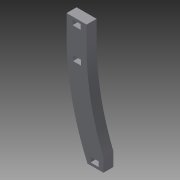
# Autodesk Inventor part: HopperFrontSupport_v2
Saved by Autodesk Inventor 2013 (Build 170138000, 138)
## iProperties
Created: 2013-01-16
Part Number: HopperFrontSupport_v2
Material: Generic
Document SubType Name: Modeling
Designer: twsass
Density: 1 g/cm^3
Mass: 47.1863 g
Surface Area: 132.222 cm^2
Volume: 47.1863 cm^3
Author: twsass
Autodesk Inventor part; units mm, degrees
ref_plane "YZ Plane" through (0, 0, 0) normal (1, 0, 0) x (0, 1, 0)
ref_plane "XZ Plane" through (0, 0, 0) normal (0, 1, 0) x (-1, 0, 0)
ref_plane "XY Plane" through (0, 0, 0) normal (0, 0, 1) x (1, 0, 0)
sketch "Sketch1" plane through (0, 0, 0) normal (0, 0, 1) x (1, 0, 0)
  circle A0 centre (0, 0) radius 292.1
  line L0 (-292.1, 0) -> (-266.7, 0)
  line L1 (-292.1, 0) -> (-317.5, 0)
  circle A1 centre (0, 0) radius 317.5
  line L2 (-317.5, 0) -> (-317.5, -127)
  line L3 (-317.5, -127) -> (-263.0464, -127)
  circle A2 centre (0, 0) radius 317.5
  dimension "d0" = 584.2
  dimension "d1" = 25.4
  dimension "d2" = 25.4
  dimension "d3" = 127
  constraints: 8 end point, 3 coincident, 2 centre point, 2 perpendicular, 2 point on circle, 1 collinear, 1 horizontal, 1 horizontal alignment, 1 vertical, 2 other
  measures "d0" diameter of A0
  measures "d1" distance of L0.start L0.end
  measures "d2" distance of L0.start L1.end
  measures "d3" distance of L1.end L2.end
extrude "Extrusion1" add sketch "Sketch1" along normal blind 12.7 contours A0 L3 A1 L1 | A1 L3 L2 picked at (-275.2864, -120.3141)
sketch "Sketch2" plane through (0, 0, 12.7) normal (0, 0, 1) x (1, 0, 0)
  line L0 (-317.5, 0) -> (-317.5, -127) projected
  line L1 (-317.5, -127) -> (-263.0464, -127) projected
  arc A0 (-292.1, 0) -> (-263.0464, -127) centre (0, 0) ccw projected
  circle A1 centre (0, 0) radius 292.1
  circle A2 centre (0, 0) radius 317.5
  line L2 (-317.5, 0) -> (-317.5, -127)
  line L3 (-317.5, -127) -> (-290.9936, -127)
  constraints: 4 end point, 2 centre point, 2 coincident, 2 point on circle, 1 collinear, 1 concentric, 1 point on line, 1 tangent
extrude "Extrusion2" cut sketch "Sketch2" against normal blind 25.4 contours A2 L1 L0
sketch "Sketch3" plane through (0, 0, 12.7) normal (0, 0, 1) x (1, 0, 0)
  arc A0 (-317.5, 0) -> (-290.9936, -127) centre (0, 0) ccw projected
  line L0 (-290.9936, -127) -> (-316.1859, -127)
  line L1 (-295.9122, -115.0749) -> (-295.9122, -127)
  line L2 (-281.9422, -117.475) -> (-276.8622, -117.475)
  line L3 (-276.8622, -117.475) -> (-276.8622, -123.825)
  line L4 (-276.8622, -123.825) -> (-287.0222, -123.825)
  line L5 (-287.0222, -123.825) -> (-287.0222, -117.475)
  line L6 (-287.0222, -117.475) -> (-281.9422, -117.475)
  line L7 (-290.9936, -127) -> (-263.0464, -127) projected
  dimension "d16" = 5.08
  dimension "d17" = 6.35
  dimension "d18" = 10.16
  dimension "d20" = 4.9186
  dimension "d33" = 13.97
  dimension "d34" = 9.525
  dimension "d35" = 8.89
  constraints: 14 end point, 2 perpendicular, 1 collinear, 1 parallel, 1 point on circle, 1 point on line
  measures "d16" distance of L2.start L2.end
  measures "d17" distance of L2.end L3.end
  measures "d18" distance of L3.end L4.end
  measures "d20" distance from line of L0.start L1
  measures "d33" distance from line of L1 L2.start
  measures "d34" distance between parallel lines of L7 L6
  measures "d35" distance between parallel lines of L1 L5
extrude "Extrusion3" cut sketch "Sketch3" against normal blind 25.4
sketch "Sketch4" plane through (0, 0, 12.7) normal (0, 0, 1) x (1, 0, 0)
  arc A0 (-317.5, 0) -> (-290.9936, -127) centre (0, 0) ccw projected
  arc A1 (-292.1, 0) -> (-263.0464, -127) centre (0, 0) ccw projected
  line L0 (-292.1, 0) -> (-317.5, 0) projected
  line L1 (-317.5, 0) -> (-317.5, 25.4)
  line L2 (-317.5, 25.4) -> (-292.1, 25.4)
  line L3 (-292.1, 25.4) -> (-292.1, 0)
  line L4 (-317.5, 0) -> (-292.1, 0)
  dimension "d24" = 25.4
  constraints: 8 end point, 3 perpendicular, 2 tangent, 1 parallel
  measures "d24" distance of L0.end L1.end
extrude "Extrusion4" add sketch "Sketch4" against normal blind 12.7
sketch "Sketch5" plane through (0, 0, 12.7) normal (0, 0, 1) x (1, 0, 0)
  line L0 (-292.1, 0) -> (-292.1, 25.4) projected
  line L1 (-292.1, 25.4) -> (-317.5, 25.4) projected
  line L2 (-317.5, 25.4) -> (-317.5, 0) projected
  line L3 (-304.8, 25.4) -> (-304.8, 22.225)
  line L4 (-304.8, 22.225) -> (-299.72, 22.225)
  line L5 (-299.72, 22.225) -> (-299.72, 15.875)
  line L6 (-299.72, 15.875) -> (-309.88, 15.875)
  line L7 (-309.88, 15.875) -> (-309.88, 22.225)
  line L8 (-309.88, 22.225) -> (-304.8, 22.225)
  dimension "d27" = 3.175
  dimension "d28" = 5.08
  dimension "d29" = 6.35
  dimension "d30" = 10.16
  constraints: 12 end point, 3 parallel, 3 perpendicular, 1 midpoint
  measures "d27" distance of L3.start L3.end
  measures "d28" distance of L3.end L4.end
  measures "d29" distance of L4.end L5.end
  measures "d30" distance of L5.end L6.end
extrude "Extrusion5" cut sketch "Sketch5" against normal blind 254
sketch "Sketch6" plane through (0, 0, 12.7) normal (0, 0, 1) x (1, 0, 0)
  line L0 (-290.9936, -127) -> (-263.0464, -127) projected
  arc A0 (-292.1, 0) -> (-263.0464, -127) centre (0, 0) ccw projected
  line L1 (-290.9936, -127) -> (-270.6736, -127)
  line L2 (-270.6736, -127) -> (-270.6736, -109.81)
  line L3 (-270.6736, -109.81) -> (-256.8603, -109.81)
  line L4 (-256.8603, -109.81) -> (-256.8603, -127)
  line L5 (-256.8603, -127) -> (-270.6736, -127)
  dimension "d36" = 20.32
  dimension "d37" = 13.8133
  constraints: 10 end point, 3 perpendicular, 1 parallel, 1 point on circle, 1 point on line
  measures "d36" distance of L0.start L1.end
  measures "d37" distance between parallel lines of L2 L4
extrude "Extrusion6" cut sketch "Sketch6" against normal blind 254 contours L2 A0 L0
sketch "Sketch7" plane through (0, 0, 12.7) normal (0, 0, 1) x (1, 0, 0)
  arc A0 (-317.5, 0) -> (-290.9936, -127) centre (0, 0) ccw projected
  line L0 (-276.8622, -117.475) -> (-276.8622, -123.825) projected
  line L1 (-317.5, 0) -> (-317.5, -127) construction
  line L2 (-317.5, -63.5) -> (-317.5, -50.8) construction
  line L3 (-317.5, -50.8) -> (-317.5, -38.1) construction
  line L4 (-317.5, -38.1) -> (-317.5, -25.4) construction
  line L5 (-317.5, -25.4) -> (-317.5, -12.7) construction
  line L6 (-317.5, 23.7649) -> (-317.5, -16.9672) construction
  line L7 (-317.5, -16.9672) -> (-180.5967, -16.9672) construction
  line L8 (-317.5, -16.9672) -> (-309.2958, -16.9672) construction
  line L9 (-309.2958, -16.9672) -> (-309.2958, -23.3172)
  line L10 (-309.2958, -23.3172) -> (-299.1358, -23.3172)
  line L11 (-299.1358, -23.3172) -> (-299.1358, -16.9672)
  line L12 (-309.2958, -16.9672) -> (-299.1358, -16.9672)
  point P0 (-317.5, 25.4)
  dimension "d59" = 8.2042
  dimension "d60" = 6.35
  dimension "d61" = 10.16
  dimension "d65" = 42.3672
  constraints: 24 end point, 7 point on line, 3 perpendicular, 2 parallel, 1 collinear, 1 midpoint, 1 tangent
  measures "d59" distance of L6.end L8.end
  measures "d60" distance of L8.end L9.end
  measures "d61" distance of L9.end L10.end
  measures "d65" distance from line of L7 point (-317.5, 25.4)
extrude "Extrusion8" cut sketch "Sketch7" against normal blind 25.4
body "Solid1"
